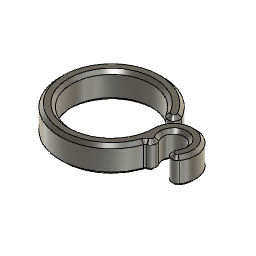
CableClip175 (Autodesk Fusion 360 design; units mm, degrees)
Autodesk Fusion 360 part; units mm, degrees
note: some values were not read from the file. Set by a fixed rule: which sketch regions a step uses.
sketch "Sketch1" plane through (0, 0, 0) normal (0, 0, 1) x (1, 0, 0)
  circle A0 centre (0, 0) radius 7.5
  circle A1 centre (0, 0) radius 9.7
  circle A2 centre (11.7, 0) radius 2
  circle A3 centre (11.7, 0) radius 4.2
  line L0 (-19.1275, 0) -> (19.1275, 0) construction
  line L1 (0, 53.4087) -> (0, -53.4087) construction
  circle A4 centre (9.1606, -1.7781) radius 1.1
  circle A5 centre (14.2394, -1.7781) radius 1.1
  circle A6 centre (7.4478, 4.3) radius 1.1
  line L2 (0, 0) -> (7.4478, 4.3) construction
  line L3 (0, 0) -> (11.7, 0) construction
  line L4 (9.1606, -1.7781) -> (11.7, 0) construction
  line L5 (14.2394, -1.7781) -> (11.7, 0) construction
  line L6 (9.1606, -1.7781) -> (14.2394, -1.7781) construction
  dimension "d5_1_1_2_1_1" = 15
  dimension "d6_1_1_2_1_1" = 2.2
  dimension "d7_1_1_2_1_1" = 4
  dimension "d9_1_1_2_1_1" = 2.2
  dimension "d17_1_1_2_1_1" = 2.2
  dimension "d18_1_1_2_1_1" = 2.2
  dimension "d23_1_1_2_1_1" = 2.2
  dimension "d32_1_1" = 110
  dimension "d34_1_1" = 90
  dimension "d36_1" = 30
  dimension "d47" = 5.0787
  constraint coincident A0.centre A1.centre
  constraint concentric A0 A1
  constraint concentric A2 A3
  constraint horizontal L0
  constraint midpoint A0.centre L0
  constraint vertical L1
  constraint midpoint A0.centre L1
  constraint tangent A0 A3
  constraint tangent A2 A4
  constraint tangent A2 A5
  constraint tangent A0 A6
  constraint coincident A6.centre L2.end
  constraint coincident A2.centre A3.centre
  constraint coincident A4.centre L4.start
  constraint coincident A5.centre L5.start
  constraint horizontal L6
  measures "d5_1_1_2_1_1" diameter of A0
  measures "d6_1_1_2_1_1" distance of A0 A1
  measures "d7_1_1_2_1_1" diameter of A2
  measures "d9_1_1_2_1_1" distance of A2 A3
  measures "d17_1_1_2_1_1" diameter of A4
  measures "d18_1_1_2_1_1" diameter of A5
  measures "d23_1_1_2_1_1" diameter of A6
  measures "d32_1_1" angle of L4 L5
  measures "d34_1_1" angle of L1 L3
  measures "d36_1" angle of L2 L3
  measures "d47" distance of A4.centre A5.centre
extrude "Extrude1" add sketch "Sketch1" along normal blind 5 contours A0 A1 A3 A6 | A1 A3 A4 | A6 | A1 A2 A3 A5 | A1 A3 A4 | A1 A4 | A1 A2 A4 | A1 A4 | A5 picked at (6.1986, 5.9178)
fillet "Fillet1" radius 0.5 1 edges at (9.2647, -2.8732, 2.5)
chamfer "Chamfer2" distance 0.6 angle 45 16 edges at (7.9978, 3.3474, 5) (-9.6544, -0.9396, 5) (9.3007, -2.9443, 5) (10.2033, -2.1285, 5) (11.7, 2, 5) (13.6084, -2.6792, 5) (12.963, 4.0056, 5) (-7.2444, -1.9411, 5) (10.2033, -2.1285, 0) (11.7, 2, 0) (13.6084, -2.6792, 0) (12.963, 4.0056, 0) (-7.2444, -1.9411, 0) (7.9978, 3.3474, 0) (-9.6544, -0.9396, 0) (9.3007, -2.9443, 0)
equation "d6_1_1_2_1_1 = ClipWall"
equation "d9_1_1_2_1_1 = ClipWall"
equation "d17_1_1_2_1_1 = ClipWall"
equation "d18_1_1_2_1_1 = ClipWall"
equation "d21_1_1_2_1_1 = Thickness"
equation "d23_1_1_2_1_1 = ClipWall"
equation "ClipWall = 2.2 mm"
equation "Thickness = 5 mm"
